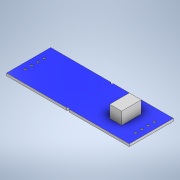
# Autodesk Inventor part: MAX485
Saved by Autodesk Inventor 2020 (Build 240168000, 168)
## iProperties
Created: 2021-10-19
Part Number: MAX485
Material: Genérico
Document SubType Name: Modeling
Designer: DANIEL
Density: 1 g/cm^3
Appearance: Valor por defecto
Author: DANIEL
Autodesk Inventor part; units mm, degrees
ref_plane "YZ Plane" through (0, 0, 0) normal (1, 0, 0) x (0, 1, 0)
ref_plane "XZ Plane" through (0, 0, 0) normal (0, 1, 0) x (-1, 0, 0)
ref_plane "XY Plane" through (0, 0, 0) normal (0, 0, 1) x (1, 0, 0)
sketch "Boceto1" plane through (0, 0, 0) normal (1, 0, 0) x (0, 1, 0)
  line L0 (0.5, 9) -> (-0.5, 9)
  line L1 (-0.5, 9) -> (-0.5, -9)
  line L2 (-0.5, -9) -> (0.5, -9)
  line L3 (0.5, -9) -> (0.5, 9)
  point P0 (0, 0)
  dimension "d0" = 1
  dimension "d1" = 18
  dimension "d2" = 9
  dimension "d3" = 0.5
  constraints: 8 end point, 2 parallel, 1 horizontal, 1 perpendicular
  measures "d0" distance between parallel lines of L1 L3
  measures "d1" distance between parallel lines of L2 L0
  measures "d2" distance from line of L0 point (0, 0)
  measures "d3" distance from line of L3 point (0, 0)
extrude "Extrusión1" add sketch "Boceto1" along normal blind 50
sketch "Boceto2" plane through (0, 0.5, 9) normal (0, 1, 0) x (1, 0, 0)
  line L0 (0, 0) -> (50, 0) projected
  line L1 (0, 18) -> (50, 18) projected
  line L2 (0, 18) -> (0, 0) projected
  line L3 (25, 0) -> (25, 18)
  line L4 (0, 0) -> (50, 0) projected
  point P0 (0, 9)
  point P1 (2.54, 5.19)
  point P2 (2.54, 7.73)
  point P3 (2.54, 10.27)
  point P4 (2.54, 12.81)
  point P5 (47.46, 5.19)
  point P6 (47.46, 7.73)
  point P7 (47.46, 10.27)
  point P8 (47.46, 12.81)
  dimension "d6" = 5.19
  dimension "d8" = 2.54
  dimension "d9" = 2.54
  dimension "d10" = 2.54
  dimension "d11" = 2.54
  constraints: 4 symmetric about line, 3 vertical alignment, 2 end point, 2 midpoint, 1 perpendicular
  measures "d6" distance from line of L0 point (2.54, 5.19)
  measures "d8" distance of point (2.54, 5.19) point (2.54, 7.73)
  measures "d9" distance of point (2.54, 7.73) point (2.54, 10.27)
  measures "d10" distance of point (2.54, 10.27) point (2.54, 12.81)
  measures "d11" distance from line of L2 point (2.54, 5.19)
hole "Agujero1" at (2.54, 0.5, 3.81) at (2.54, 0.5, 1.27) at (2.54, 0.5, -1.27) at (2.54, 0.5, -3.81) at (25, 0.5, 9) at (25, 0.5, -9) at (47.46, 0.5, -3.81) at (47.46, 0.5, -1.27) at (47.46, 0.5, 1.27) at (47.46, 0.5, 3.81) direction (0, -1, 0) diameter 0.9 end through all
sketch "Boceto3" plane through (0, 0.5, 9) normal (0, 1, 0) x (1, 0, 0)
  line L0 (37.0371, 5) -> (41.9064, 5)
  line L1 (41.9064, 5) -> (41.9064, 13)
  line L2 (41.9064, 13) -> (37.0371, 13)
  line L3 (37.0371, 13) -> (37.0371, 5)
  line L4 (25.45, 0) -> (50, 0) projected
  line L5 (25.45, 18) -> (50, 18) projected
  point P0 (0, 9)
  dimension "d19" = 5
  dimension "d20" = 5
  constraints: 8 end point, 2 parallel, 1 horizontal, 1 perpendicular
  measures "d19" distance between parallel lines of L4 L0
  measures "d20" distance between parallel lines of L5 L2
extrude "Extrusión2" add sketch "Boceto3" along normal blind 5
